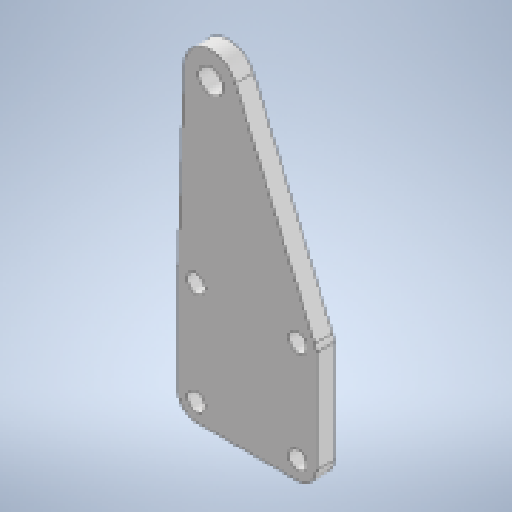
# Autodesk Inventor part: Uchwyt_na_enkoder
Saved by Autodesk Inventor 2023 (Build 270158000, 158)
## iProperties
Created: 2023-02-28
Part Number: Uchwyt_na_enkoder
Material: Ogólny
Document SubType Name: Modeling
Designer: Kamil
Density: 1 g/cm^3
Appearance: Domyślna
Author: Kamil
Autodesk Inventor part; units mm, degrees
ref_plane "YZ Plane" through (0, 0, 0) normal (1, 0, 0) x (0, 1, 0)
ref_plane "XZ Plane" through (0, 0, 0) normal (0, 1, 0) x (-1, 0, 0)
ref_plane "XY Plane" through (0, 0, 0) normal (0, 0, 1) x (1, 0, 0)
sketch "Szkic1" plane through (0, 0, 0) normal (0, 0, 1) x (1, 0, 0)
  arc A0 (-8.5, 11.5) -> (-11.5, 8.5) centre (-8.5, 8.5) ccw projected
  line L0 (-11.5, 8.5) -> (-11.5, -8.5) projected
  arc A1 (-11.5, -8.5) -> (-8.5, -11.5) centre (-8.5, -8.5) ccw projected
  line L1 (-8.5, -11.5) -> (8.5, -11.5) projected
  arc A2 (8.5, -11.5) -> (11.5, -8.5) centre (8.5, -8.5) ccw projected
  line L2 (11.5, -8.5) -> (11.5, 8.5) projected
  arc A3 (11.5, 8.5) -> (8.5, 11.5) centre (8.5, 8.5) ccw projected
  line L3 (8.5, 11.5) -> (-8.5, 11.5) projected
  circle A4 centre (2.14, 6.5) radius 0.5 projected
  circle A5 centre (-0.4, 6.5) radius 0.5 projected
  circle A6 centre (-1.58, -6.5) radius 0.5 projected
  circle A7 centre (0.96, -6.5) radius 0.5 projected
  circle A8 centre (3.5, -6.5) radius 0.5 projected
  circle A9 centre (-4.12, -6.5) radius 0.5 projected
  circle A10 centre (-8.5, 8.5) radius 1.5 projected
  circle A11 centre (8.5, 8.5) radius 1.5 projected
  circle A12 centre (8.5, -8.5) radius 1.5 projected
  circle A13 centre (-8.5, -8.5) radius 1.5 projected
  circle A14 centre (-2.94, 6.5) radius 0.5 projected
  circle A15 centre (-8.5, -8.5) radius 3
  circle A16 centre (-8.5, 8.5) radius 3
  circle A17 centre (8.5, -8.5) radius 3
  circle A18 centre (8.5, 8.5) radius 3
  circle A19 centre (-6.0386, 38.934) radius 2 projected
  arc A20 (-9.5915, 35.416) -> (-1.5869, 36.6574) centre (-6.0386, 38.934) ccw projected
  arc A21 (-9.5915, 35.416) -> (-15.0494, 36.5208) centre (-13.1444, 31.8979) ccw projected
  arc A22 (3.2799, 39.3636) -> (-1.5869, 36.6574) centre (2.8647, 34.3809) ccw projected
  circle A23 centre (-6.0386, 38.934) radius 2 projected
  arc A24 (-15.0494, 36.5208) -> (-15.1665, -36.4723) centre (0, 0) ccw projected
  arc A25 (3.4887, -39.3456) -> (3.2799, 39.3636) centre (0, 0) ccw projected
  arc A26 (3.5329, -39.8437) -> (3.3214, 39.8619) centre (0, 0) ccw
  arc A27 (3.3214, 39.8619) -> (-2.0321, 36.8851) centre (2.8647, 34.3809) ccw
  arc A28 (-9.2362, 35.7678) -> (-2.0321, 36.8851) centre (-6.0386, 38.934) ccw
  arc A29 (-9.2362, 35.7678) -> (-15.2399, 36.9831) centre (-13.1444, 31.8979) ccw
  arc A30 (-15.2399, 36.9831) -> (-15.3585, -36.9339) centre (0, 0) ccw
  circle A31 centre (-6.0386, 38.934) radius 4.5
  line L4 (13.6965, 37.6445) -> (-11.8601, 45.4046)
  line L5 (-24.522, 31.6817) -> (-6.4094, 44.1408)
  line L6 (15.4037, -0.0931) -> (-1.1009, 38.8173)
  line L7 (-11.4685, 9.5445) -> (-9.9618, 57.2756)
  line L8 (-1.1009, 38.8173) -> (-1.8958, 40.6913)
  line L9 (-11.4685, 9.5445) -> (-11.5, 8.5)
  point P0 (0, 0)
  point P1 (-10.5363, 39.076)
  point P2 (11.2618, 9.6715)
  dimension "d2" = 6
  dimension "d1" = 6
  dimension "d3" = 6
  dimension "d4" = 6
  dimension "d6" = 0.5
  constraints: 12 end point, 10 point on circle, 8 centre point, 4 coincident, 4 tangent, 1 horizontal alignment, 1 point on line, 14 other
  measures "d1" diameter of A15
  measures "d3" diameter of A17
  measures "d4" diameter of A18
  measures "d6" radial gap between concentric circles of A20 A28
extrude "Wyciągnięcie proste1" add sketch "Szkic1" along normal blind 3 contours A16 A0 | L9 L7 A21 A20 A22 L6 A3 A18 L2 A17 L1 A15 L0 | A15 A1 | L7 A29 A28 A27 L6 A22 A20 A21 | A17 A2 | L7 A31 A29 | A31 A28 | A18 A3 | A31 L8 L6 A27 | A4 | A5 | A6 | A7 | A8 | A9 | A14
sketch "Szkic2" plane through (0, 0, 0) normal (0, 0, -1) x (-1, 0, 0)
  line L0 (-8.5, 11.5) -> (8.5, 11.5) projected
  arc A0 (11.5, 8.5) -> (8.5, 11.5) centre (8.5, 8.5) ccw projected
  arc A1 (11.5, 8.5) -> (8.5, 11.5) centre (8.5, 8.5) ccw projected
  line L1 (8.5, 11.5) -> (-8.5, 11.5) projected
  arc A2 (-8.5, 11.5) -> (-11.5, 8.5) centre (-8.5, 8.5) ccw projected
  line L2 (-11.5, 8.5) -> (-11.5, -8.5) projected
  arc A3 (-11.5, -8.5) -> (-8.5, -11.5) centre (-8.5, -8.5) ccw projected
  line L3 (-8.5, -11.5) -> (8.5, -11.5) projected
  arc A4 (8.5, -11.5) -> (11.5, -8.5) centre (8.5, -8.5) ccw projected
  line L4 (11.5, -8.5) -> (11.5, 8.5) projected
  line L5 (6.9, 0.37) -> (6.9, -0.63) projected
  line L6 (6.9, -0.63) -> (5.02, -0.63) projected
  line L7 (5.02, -0.63) -> (5.02, 0.37) projected
  line L8 (5.02, 0.37) -> (6.9, 0.37) projected
  line L9 (6.9, 3.37) -> (6.9, 2.37) projected
  line L10 (6.9, 2.37) -> (5.02, 2.37) projected
  line L11 (5.02, 2.37) -> (5.02, 3.37) projected
  line L12 (5.02, 3.37) -> (6.9, 3.37) projected
  line L13 (6.9, -2.63) -> (6.9, -3.63) projected
  line L14 (6.9, -3.63) -> (5.02, -3.63) projected
  line L15 (5.02, -3.63) -> (5.02, -2.63) projected
  line L16 (5.02, -2.63) -> (6.9, -2.63) projected
  line L17 (-6.22, -3.5) -> (-6.22, -4.5) projected
  line L18 (-6.22, -4.5) -> (-8.1, -4.5) projected
  line L19 (-8.1, -4.5) -> (-8.1, -3.5) projected
  line L20 (-8.1, -3.5) -> (-6.22, -3.5) projected
  line L21 (-6.22, 3.5) -> (-6.22, 2.5) projected
  line L22 (-6.22, 2.5) -> (-8.1, 2.5) projected
  line L23 (-8.1, 2.5) -> (-8.1, 3.5) projected
  line L24 (-8.1, 3.5) -> (-6.22, 3.5) projected
  line L25 (-6.22, 0) -> (-6.22, -1) projected
  line L26 (-6.22, -1) -> (-8.1, -1) projected
  line L27 (-8.1, -1) -> (-8.1, 0) projected
  line L28 (-8.1, 0) -> (-6.22, 0) projected
  line L29 (2.5, -2.1) -> (-2.5, -2.1) projected
  line L30 (-2.5, -2.1) -> (-2.5, 2.1) projected
  line L31 (-2.5, 2.1) -> (2.5, 2.1) projected
  line L32 (2.5, 2.1) -> (2.5, -2.1) projected
  circle A5 centre (-2.14, 6.5) radius 0.5 projected
  circle A6 centre (0.4, 6.5) radius 0.5 projected
  circle A7 centre (1.58, -6.5) radius 0.5 projected
  circle A8 centre (-0.96, -6.5) radius 0.5 projected
  circle A9 centre (-3.5, -6.5) radius 0.5 projected
  circle A10 centre (4.12, -6.5) radius 0.5 projected
  circle A11 centre (8.5, 8.5) radius 1.5 projected
  circle A12 centre (-8.5, 8.5) radius 1.5 projected
  circle A13 centre (-8.5, -8.5) radius 1.5 projected
  circle A14 centre (8.5, -8.5) radius 1.5 projected
  circle A15 centre (2.94, 6.5) radius 0.5 projected
  line L33 (10.5363, 39.076) -> (11.4685, 9.5445) projected
  arc A16 (10.5363, 39.076) -> (1.8958, 40.6913) centre (6.0386, 38.934) ccw projected
  line L34 (-11.2618, 9.6715) -> (1.8958, 40.6913) projected
  arc A17 (-11.2618, 9.6715) -> (-11.5, 8.5) centre (-8.5, 8.5) ccw projected
  line L35 (-11.5, -8.5) -> (-11.5, 8.5) projected
  arc A18 (-11.5, -8.5) -> (-8.5, -11.5) centre (-8.5, -8.5) ccw projected
  line L36 (8.5, -11.5) -> (-8.5, -11.5) projected
  arc A19 (8.5, -11.5) -> (11.5, -8.5) centre (8.5, -8.5) ccw projected
  line L37 (11.5, 8.5) -> (11.5, -8.5) projected
  line L38 (11.4685, 9.5445) -> (11.5, 8.5) projected
  circle A20 centre (-8.5, -8.5) radius 1.5 projected
  circle A21 centre (8.5, -8.5) radius 1.5 projected
  circle A22 centre (-8.5, 8.5) radius 1.5 projected
  circle A23 centre (8.5, 8.5) radius 1.5 projected
  circle A24 centre (6.0386, 38.934) radius 2 projected
  line L39 (0, 11.5) -> (0, 14)
  line L40 (0, 14) -> (-18.1908, 14)
  line L41 (-18.1908, 14) -> (-18.1908, 37.174)
  line L42 (-18.1908, 37.174) -> (0, 37.174)
  line L43 (0, 37.174) -> (0, 14)
  line L44 (0, 14) -> (41.2236, 14)
  line L45 (41.2236, 14) -> (41.2236, 46.0216)
  line L46 (41.2236, 46.0216) -> (0, 46.0216)
  line L47 (0, 46.0216) -> (0, 14)
  point P0 (0, 0)
  point P1 (-9.4258, 14)
  point P2 (11.3279, 14)
  dimension "d9" = 2.5
  constraints: 18 end point, 4 parallel, 3 perpendicular, 2 horizontal, 1 midpoint
  measures "d9" distance of L39.start L39.end
extrude "Wyciągnięcie proste2" add sketch "Szkic2" along normal blind 9 contours L40 L34 L43 | L43 L34 A16 L33 L44
sketch "Szkic3" plane through (0, 0, -9) normal (0, 0, -1) x (-1, 0, 0)
  arc A0 (15.1665, -36.4723) -> (15.0494, 36.5208) centre (0, 0) ccw projected
  arc A1 (15.0494, 36.5208) -> (9.5915, 35.416) centre (13.1444, 31.8979) ccw projected
  arc A2 (1.5869, 36.6574) -> (-3.2799, 39.3636) centre (-2.8647, 34.3809) ccw projected
  arc A3 (10.5363, 39.076) -> (1.8958, 40.6913) centre (6.0386, 38.934) ccw projected
  arc A4 (1.5869, 36.6574) -> (9.5915, 35.416) centre (6.0386, 38.934) ccw projected
  arc A5 (15.0494, 36.5208) -> (9.5915, 35.416) centre (13.1444, 31.8979) ccw projected
  arc A6 (1.5869, 36.6574) -> (-3.2799, 39.3636) centre (-2.8647, 34.3809) ccw projected
  arc A7 (1.5869, 36.6574) -> (-3.2799, 39.3636) centre (-2.8647, 34.3809) ccw projected
  arc A8 (1.5869, 36.6574) -> (9.5915, 35.416) centre (6.0386, 38.934) ccw projected
  circle A9 centre (6.0386, 38.934) radius 4.5
  point P0 (0, 0)
  point P1 (10.5363, 39.076)
  constraints: 1 centre point, 1 coincident
ref_plane "Płaszczyzna konstrukcyjna1" through (-55.4425, -46.0546, -29) normal (0, 0, 1) x (0.9999995, 0.0009905, 0)
extrude "Wyciągnięcie proste3" add sketch "Szkic3" along normal up to surface (20 mm away)
sketch "Szkic4" plane through (-11.5, -8.5, 0) normal (-1, 0, 0) x (0, 0, 1)
  line L0 (0, 17) -> (0, 0) projected
  line L1 (0, 0) -> (3, 0) projected
  line L2 (3, 17) -> (3, 0) projected
  line L3 (0, 17) -> (3, 17) projected
  line L4 (0, 22.5) -> (0, 18.0445) projected
  line L5 (0, 18.0445) -> (3, 18.0445) projected
  line L6 (3, 47.576) -> (3, 18.0445) projected
  line L7 (3, 47.576) -> (-9, 47.576) projected
  line L8 (-9, 22.5) -> (-9, 47.576) projected
  line L9 (0, 22.5) -> (-9, 22.5) projected
  line L10 (0, 18.0445) -> (0, 17) projected
  line L11 (0, 17) -> (3, 17) projected
  line L12 (3, 18.0445) -> (3, 17) projected
  line L13 (0, 18.0445) -> (3, 18.0445) projected
  line L14 (-29, 51.934) -> (-29, 42.934) projected
  line L15 (3, 47.576) -> (-9, 47.576) projected
  line L16 (3, 49.1913) -> (3, 47.576) projected
  line L17 (-9, 49.1913) -> (3, 49.1913) projected
  line L18 (-9, 47.576) -> (-9, 49.1913) projected
  line L19 (-29, 42.934) -> (-9, 42.934) projected
  line L20 (-29, 51.934) -> (3, 51.934) projected
  line L21 (3, 22.5) -> (-17.3354, 68.6705)
  line L22 (0, 22.5) -> (-9, 42.934)
  line L23 (3, 49.1913) -> (3, 51.934)
  point P0 (0, 8.5)
  point P1 (-9.964, 51.934)
  constraints: 6 end point, 1 parallel, 1 point on line, 1 vertical
extrude "Wyciągnięcie proste4" cut sketch "Szkic4" against normal through all contours L9 L8 L22 | L21 L7 L6 | L7 L21 L17 L16 | L17 L21 L20 L23
sketch "Szkic5" plane through (-6.0386, 38.934, -29) normal (0, 0, -1) x (-1, 0, 0)
  circle A0 centre (0, 0) radius 4.5 projected
  circle A1 centre (0, 0) radius 2 projected
  circle A2 centre (0, 0) radius 2.25
  point P0 (-6.0386, -38.934)
  dimension "d16" = 4.5
  constraints: 1 centre point, 1 coincident
  measures "d16" diameter of A2
extrude "Wyciągnięcie proste5" cut sketch "Szkic5" against normal through all contours A1 | A2
sketch "Szkic6" plane through (0, 0, -9) normal (0, 0, -1) x (-1, 0, 0)
  line L0 (-0.7583, 34.434) -> (6.0386, 34.434) projected
  arc A0 (1.8958, 40.6913) -> (6.0386, 34.434) centre (6.0386, 38.934) ccw projected
  line L1 (1.8958, 40.6913) -> (-0.7583, 34.434) projected
  line L2 (6.0386, 34.434) -> (10.6829, 34.434) projected
  line L3 (10.6829, 34.434) -> (10.5363, 39.076) projected
  arc A1 (6.0386, 34.434) -> (10.5363, 39.076) centre (6.0386, 38.934) ccw projected
  point P0 (0, 0)
extrude "Wyciągnięcie proste6" add sketch "Szkic6" along normal blind 3
fillet "Zaokrąglenie5" radius 15 1 edges at (-0.951, 14, 0)
sketch "Szkic7" plane through (0, 0, 3) normal (0, 0, 1) x (1, 0, 0)
  circle A0 centre (-6.0386, 38.934) radius 2.25 projected
  circle A1 centre (-6.0386, 38.934) radius 2.9
  point P0 (0, 0)
  dimension "d26" = 5.8
  constraints: 1 centre point, 1 coincident
  measures "d26" diameter of A1
extrude "Wyciągnięcie proste7" cut sketch "Szkic7" against normal blind 29 contours A0 | A1
fillet "Zaokrąglenie6" radius 15 1 edges at (-0.951, 14, 3)
